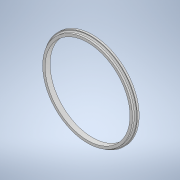
# Autodesk Inventor part: DriftGummisPvcKlebestütze
Saved by Autodesk Inventor 2021 (Build 250183000, 183)
## iProperties
Created: 2021-05-26
Part Number: DriftGummisPvcKlebestütze
Material: Generisch
Document SubType Name: Modeling
Designer: Lars-Ole
Density: 1 g/cm^3
Appearance: Vorgabe
Author: Lars-Ole
Autodesk Inventor part; units mm, degrees
ref_plane "YZ Plane" through (0, 0, 0) normal (1, 0, 0) x (0, 1, 0)
ref_plane "XZ Plane" through (0, 0, 0) normal (0, 1, 0) x (-1, 0, 0)
ref_plane "XY Plane" through (0, 0, 0) normal (0, 0, 1) x (1, 0, 0)
sketch "Skizze1" plane through (0, 0, 0) normal (0, 1, 0) x (-1, 0, 0)
  line L0 (0, -1.6) -> (0, 9.6) projected
  line L1 (-69, 0) -> (-69, 8)
  line L2 (-69, 8) -> (-73, 8)
  line L3 (-76, 0) -> (-69, 0)
  line L4 (-73, 8) -> (-73, 3)
  line L5 (-73, 3) -> (-76, 3)
  line L6 (-76, 3) -> (-76, 0)
  point P0 (0, 0)
  dimension "d0" = 152
  dimension "d1" = 8
  dimension "d2" = 7
  dimension "d3" = 4
  dimension "d4" = 3
  constraints: 12 end point, 3 perpendicular, 2 vertical, 1 parallel, 1 point on line
  measures "d0" diameter of L3.start L0
  measures "d1" distance of L1.start L1.end
  measures "d2" distance from line of L3.start L1
  measures "d3" distance of L1.end L2.end
  measures "d4" distance of L5.end L3.start
revolve "Umdrehung1" add sketch "Skizze1" angle 360 about axis through (0, 0, -10) along (0, 0, 1)
fillet "Rundung1" radius 2 1 edges at (-73, 0, 3)
